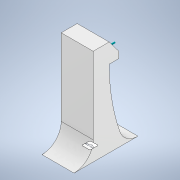
# Autodesk Inventor part: Clipje
Saved by Autodesk Inventor 2022 (Build 260153000, 153)
## iProperties
Created: 2022-02-17
Part Number: Clipje
Material: ABS Plastic
Document SubType Name: Modeling
Designer: woutr
Density: 1.06 g/cm^3
Appearance: Smooth - White
Author: woutr
Autodesk Inventor part; units mm, degrees
ref_plane "YZ Plane" through (0, 0, 0) normal (1, 0, 0) x (0, 1, 0)
ref_plane "XZ Plane" through (0, 0, 0) normal (0, 1, 0) x (-1, 0, 0)
ref_plane "XY Plane" through (0, 0, 0) normal (0, 0, 1) x (1, 0, 0)
sketch "Sketch1" plane through (0, 0, 0) normal (1, 0, 0) x (0, 1, 0)
  line L0 (3, 0) -> (15, 0)
  line L1 (15, 0) -> (15, -2.5)
  line L2 (15, -2.5) -> (13, -4)
  line L3 (13, -4) -> (12, -4)
  line L4 (12, -4) -> (12, -2.5)
  line L5 (0, -4) -> (0, 0)
  arc A0 (12, -2.5) -> (2.027, -4.1622) centre (12, -33.25) ccw
  line L6 (0, 3) -> (0, 0)
  arc A1 (0, 3) -> (3, 0) centre (3, 3) ccw
  line L7 (0, -4) -> (0, -7)
  arc A2 (2.027, -4.1622) -> (0, -7) centre (3, -7) ccw
  dimension "d0" = 12
  dimension "d1" = 4
  dimension "d2" = 1.5
  dimension "d3" = 3
  dimension "d4" = 2.5
  dimension "d5" = 1
  dimension "d15" = 3
  dimension "d17" = 3
  dimension "d18" = 3
  constraints: 16 end point, 6 point on circle, 4 tangent, 3 centre point, 2 horizontal alignment, 2 parallel, 2 perpendicular, 2 vertical, 1 horizontal, 1 point on line
  measures "d0" distance between parallel lines of L4 L5
  measures "d1" distance of L5.start L5.end
  measures "d2" distance of L3.end L4.end
  measures "d3" distance between parallel lines of L1 L4
  measures "d4" distance from line of L0 L4.end
  measures "d5" distance of L2.end L3.end
  measures "d15" radius of A1
  measures "d17" radius of A2
  measures "d18" distance of L5.start L7.end
extrude "Extrusion1" add sketch "Sketch1" along normal blind 5
body "Solid1"
